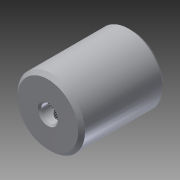
# Autodesk Inventor part: ZACMEFlexCoupler
Saved by Autodesk Inventor 2015 SP1 (Build 190203100, 203)
## iProperties
Category: Hardware
Created: 2014-01-02
Part Number: ZACMEFlexCoupler
Material: Aluminum 6061
Document SubType Name: Modeling
Designer: Jack
Density: 2.71 g/cm^3
Appearance: Aluminum - Flat
Mass: 18.341 g
Surface Area: 27.9429 cm^2
Volume: 6.76789 cm^3
Vendor: MakersToolWorks
Author: Jack
Title: Z Axis Flex Coupler
Autodesk Inventor part; units mm, degrees
ref_plane "YZ Plane" through (0, 0, 0) normal (1, 0, 0) x (0, 1, 0)
ref_plane "XZ Plane" through (0, 0, 0) normal (0, 1, 0) x (-1, 0, 0)
ref_plane "XY Plane" through (0, 0, 0) normal (0, 0, 1) x (1, 0, 0)
sketch "Sketch1" plane through (0, 0, 0) normal (0, 1, 0) x (-1, 0, 0)
  circle A0 centre (0, 0) radius 10
  dimension "d0" = 20
  constraints: 1 centre point, 1 coincident
  measures "d0" diameter of A0
extrude "Extrusion1" add sketch "Sketch1" along normal blind 25
sketch "Sketch2" plane through (0, 25, 0) normal (0, 1, 0) x (1, 0, 0)
  circle A0 centre (0, 0) radius 10 projected
  circle A1 centre (0, 0) radius 2.5
  dimension "d3" = 5
  constraints: 1 centre point, 1 coincident
  measures "d3" diameter of A1
extrude "Extrusion2" cut sketch "Sketch2" against normal blind 14 contours A1
sketch "Sketch3" plane through (0, 0, 0) normal (0, -1, 0) x (1, 0, 0)
  circle A0 centre (0, 0) radius 10 projected
  circle A1 centre (0, 0) radius 2.5
  dimension "d6" = 5
  constraints: 1 centre point, 1 coincident
  measures "d6" diameter of A1
extrude "Extrusion3" cut sketch "Sketch3" against normal blind 11 contours A1
chamfer "Chamfer1" distance 1 angle 45 2 edges at (10, 25, 0) (10, 0, 0)
chamfer "Chamfer2" distance 0.5 angle 45 2 edges at (-2.5, 25, 0) (-2.5, 0, 0)
sketch "Sketch4" plane through (0, 25, 0) normal (0, 1, 0) x (1, 0, 0)
  circle A0 centre (0, 0) radius 9 projected
  circle A1 centre (0, 0) radius 3 projected
  circle A2 centre (0, 0) radius 10 projected
  line L0 (-10, 0) -> (10, 0) construction
  line L1 (0, 0) -> (-9.6593, -2.5882) construction
  point P0 (0, 10)
  point P1 (-9.6593, -2.5882)
  dimension "d28" = 15
  constraints: 4 end point, 4 point on circle, 1 coincident, 1 horizontal, 1 midpoint, 1 vertical alignment
  measures "d28" angle of L0 L1
ref_plane "Work Plane1" through (0, 25, -10) normal (0, 0, -1) x (-1, 0, 0)
ref_plane "Work Plane3" through (-9.6593, 25, 2.5882) normal (-0.9659258, 0, 0.258819) x (0, -1, 0)
sketch "Sketch5" plane through (0, 25, -10) normal (0, 0, -1) x (-1, 0, 0)
  line L0 (10, -1) -> (-10, -1) projected
  line L1 (-10, -24) -> (10, -24) projected
  line L2 (-10, -24) -> (-10, -1) projected
  line L3 (10, -24) -> (10, -1) projected
  circle A0 centre (0, -4.5) radius 2
  circle A1 centre (0, -20.5) radius 2
  line L4 (-9, 0) -> (9, 0) projected
  line L5 (9, -25) -> (-9, -25) projected
  point P0 (0, -25)
  point P1 (0, -1)
  dimension "d16" = 4
  dimension "d17" = 4
  dimension "d18" = 4.5
  dimension "d19" = 4.5
  constraints: 2 centre point, 2 vertical alignment, 1 midpoint
  measures "d16" diameter of A0
  measures "d17" diameter of A1
  measures "d18" distance from line of L5 A1.centre
  measures "d19" distance from line of L4 A0.centre
extrude "Extrusion4" cut sketch "Sketch5" against normal blind 8.75 contours A0 | A1
sketch "Sketch6" plane through (-9.6593, 25, 2.5882) normal (-0.9659258, 0, 0.258819) x (0, -1, 0)
  circle A0 centre (4.5, 0) radius 2
  line L0 (24, -10) -> (1, -10) projected
  line L1 (24, 10) -> (1, 10) projected
  line L2 (25, 9) -> (25, -9) projected
  line L3 (0, -9) -> (0, 9) projected
  circle A1 centre (20.5, 0) radius 2
  point P0 (25, 0)
  point P1 (0, 0)
  dimension "d22" = 4
  dimension "d23" = 4
  dimension "d24" = 4.5
  dimension "d25" = 4.5
  constraints: 2 centre point, 2 horizontal alignment, 1 midpoint
  measures "d22" diameter of A0
  measures "d23" diameter of A1
  measures "d24" distance from line of L2 A1.centre
  measures "d25" distance from line of A0.centre L3
extrude "Extrusion5" cut sketch "Sketch6" against normal blind 8.75
thread "Thread1" size "M4x0.7" class "6H" standard "ANSI Metric M Profile" full length
thread "Thread2" size "M4x0.7" class "6H" standard "ANSI Metric M Profile" full length
thread "Thread3" size "M4x0.7" class "6H" standard "ANSI Metric M Profile" full length
thread "Thread4" size "M4x0.7" class "6H" standard "ANSI Metric M Profile" full length
body "Solid1"
